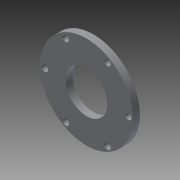
# Autodesk Inventor part: Stator Front
Saved by Autodesk Inventor 2018.2 (Build 222227000, 227)
## iProperties
Created: 2018-02-06
Part Number: Stator Front
Material: Generic
Document SubType Name: Modeling
Designer: Rus
Density: 1 g/cm^3
Appearance: Default
Author: Rus
Autodesk Inventor part; units mm, degrees
ref_plane "YZ Plane" through (0, 0, 0) normal (1, 0, 0) x (0, 1, 0)
ref_plane "XZ Plane" through (0, 0, 0) normal (0, 1, 0) x (-1, 0, 0)
ref_plane "XY Plane" through (0, 0, 0) normal (0, 0, 1) x (1, 0, 0)
sketch "Sketch1" plane through (0, 0, 0) normal (0, 0, 1) x (1, 0, 0)
  circle A0 centre (0, 0) radius 46.5667
  circle A1 centre (0, 0) radius 19.05
  dimension "d0" = 93.1333
  dimension "d1" = 38.1
  constraints: 2 centre point, 2 coincident
  measures "d0" diameter of A0
  measures "d1" diameter of A1
extrude "Extrusion1" add sketch "Sketch1" along normal blind 6.35
sketch "Sketch2" plane through (0, 0, 6.35) normal (0, 0, 1) x (1, 0, 0)
  line L0 (21.1667, 36.6617) -> (42.3333, 0) construction
  line L1 (42.3333, 0) -> (21.1667, -36.6617) construction
  line L2 (21.1667, -36.6617) -> (-21.1667, -36.6617) construction
  line L3 (-21.1667, -36.6617) -> (-42.3333, 0) construction
  line L4 (-42.3333, 0) -> (-21.1667, 36.6617) construction
  line L5 (-21.1667, 36.6617) -> (21.1667, 36.6617) construction
  line L6 (-21.1667, 36.6617) -> (-23.2833, 40.3279) construction
  circle A0 centre (0, 0) radius 46.5667 construction
  dimension "d4" = 4.2333
  constraints: 14 end point, 1 coincident, 1 horizontal, 16 other
  measures "d4" distance of L4.end L6.end
hole "Hole1" at (-21.1667, 36.6617, 6.35) at (-42.3333, 0, 6.35) at (-21.1667, -36.6617, 6.35) at (42.3333, 0, 6.35) at (21.1667, -36.6617, 6.35) at (21.1667, 36.6617, 6.35) direction (0, 0, -1) diameter 6 end through all
body "Solid1"
